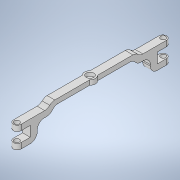
# Autodesk Inventor part: Балка рулевого управления
Saved by Autodesk Inventor 2020 (Build 240168000, 168)
## iProperties
Created: 2021-03-21
Part Number: Балка рулевого управления
Material: Типовые
Document SubType Name: Modeling
Designer: Антон
Density: 1 g/cm^3
Appearance: По умолчанию
Author: Антон
Autodesk Inventor part; units mm, degrees
ref_plane "YZ Plane" through (0, 0, 0) normal (1, 0, 0) x (0, 1, 0)
ref_plane "XZ Plane" through (0, 0, 0) normal (0, 1, 0) x (-1, 0, 0)
ref_plane "XY Plane" through (0, 0, 0) normal (0, 0, 1) x (1, 0, 0)
sketch "Эскиз1" plane through (0, 0, 0) normal (0, 1, 0) x (-1, 0, 0)
  line L0 (0, 0) -> (5.5, 0)
  line L1 (5.5, 0) -> (5.5, -55.05)
  line L2 (5.5, -55.05) -> (0, -55.05)
  line L3 (0, -55.05) -> (0, 0)
  line L4 (2.75, 0) -> (2.75, -2.5)
  circle A0 centre (2.75, -2.5) radius 1.85
  dimension "d0" = 5.5
  dimension "d1" = 55.05
  dimension "d4" = 2.5
  dimension "d5" = 3.7
  constraints: 10 end point, 2 parallel, 1 centre point, 1 coincident, 1 horizontal, 1 midpoint, 1 perpendicular, 1 vertical
  measures "d0" distance of L1.end L2.end
  measures "d1" distance of L0.end L1.end
  measures "d4" distance of L4.start L4.end
  measures "d5" diameter of A0
extrude "Выдавливание1" add sketch "Эскиз1" along normal blind 4
fillet "Сопряжение1" radius 2.75 2 edges at (0, 2, 0) (-5.5, 2, 0)
sketch "Эскиз2" plane through (0, 4, 0) normal (0, 1, 0) x (1, 0, 0)
  line L0 (0, 2.75) -> (0, 55.05) projected
  line L1 (-5.5, 55.05) -> (0, 55.05)
  line L2 (0, 55.05) -> (0, 9.4)
  line L3 (0, 9.4) -> (-5.5, 9.4)
  line L4 (-5.5, 9.4) -> (-5.5, 55.05)
  point P0 (0, 0)
  dimension "d7" = 45.65
  dimension "d45" = 52.3
  constraints: 8 end point, 2 parallel, 1 horizontal, 1 perpendicular, 1 point on line
  measures "d7" distance of L1.end L2.end
  measures "d45" distance of L0.start L0.end
extrude "Выдавливание2" add sketch "Эскиз2" along normal blind 3.7
mirror "Зеркальное отражение3" about plane through (-2.75, 7.7, -32.225) normal (0, 1, 0)
sketch "Эскиз8" plane through (0, 0, -2.75) normal (1, 0, 0) x (0, 0, -1)
  line L0 (0, 0) -> (52.3, 0) projected
  line L1 (52.3, 0) -> (11.65, 0)
  line L2 (11.65, 0) -> (11.65, 15)
  line L3 (11.65, 15) -> (52.3, 15)
  line L4 (52.3, 15) -> (52.3, 0)
  line L5 (6.65, 4) -> (6.65, 11.4) projected
  line L6 (11.65, 15) -> (21.65, 15)
  line L7 (21.65, 15) -> (21.65, 11)
  line L8 (21.65, 11) -> (11.65, 11)
  line L9 (11.65, 11) -> (11.65, 15)
  point P0 (-2.75, 0)
  dimension "d35" = 40.65
  dimension "d36" = 15
  dimension "d52" = 45.65
  dimension "d60" = 10
  dimension "d61" = 4
  constraints: 14 end point, 3 horizontal, 3 parallel, 2 perpendicular, 3 other
  measures "d35" distance of L2.end L4.start
  measures "d36" distance of L1.end L2.end
  measures "d52" distance between parallel lines of L4 L5
  measures "d60" distance of L7.end L8.end
  measures "d61" distance of L6.end L7.end
extrude "Выдавливание6" cut sketch "Эскиз8" against normal through all contours L2 L8 L7 L3 L4 L0
sketch "Эскиз13" plane through (-5.5, 15.4, -55.05) normal (0, 1, 0) x (1, 0, 0)
  line L0 (0, 0) -> (0, -30.65) projected
  line L1 (5.5, 0) -> (0, 0) projected
  line L2 (5.5, -30.65) -> (5.5, 0) projected
  line L3 (5.5, -30.65) -> (0, -30.65) projected
  point P0 (5.5, -55.05)
extrude "Выдавливание11" add sketch "Эскиз13" along normal blind 3
mirror "Зеркальное отражение6" about plane through (0, 0, -55.05) normal (0, 0, -1)
fillet "Сопряжение5" radius 5 12 edges at (-2.75, 0, -14.4) (-2.75, 0, -95.7) (-2.75, 11, -14.4) (-2.75, 11, -24.4) (-2.75, 15, -24.4) (-2.75, 11, -95.7) (-2.75, 11, -85.7) (-2.75, 15, -85.7) (-2.75, 18.4, -24.4) (-2.75, 18.4, -85.7) (-2.75, 15.4, -24.4) (-2.75, 15.4, -85.7)
sketch "Эскиз9" plane through (-2.75, 18.4, -2.75) normal (0, 1, 0) x (1, 0, 0)
  line L0 (2.75, 0) -> (2.75, 21.65) projected
  line L1 (2.75, 52.3) -> (-2.75, 52.3)
  line L2 (-2.75, 21.65) -> (-2.75, 0) projected
  circle A0 centre (0, 52.3) radius 4
  point P0 (2.75, -2.75)
  point P1 (2.75, 104.6)
  point P2 (-2.75, 104.6)
  point P3 (-2.75, 0)
  point P4 (60.3162, 64.5588)
  point P5 (-2.1213, 2.1213)
  point P6 (2.75, 11.65)
  point P7 (-2.75, 11.65)
  point P8 (-2.75, 21.65)
  dimension "d46" = 8
  constraints: 2 end point, 1 centre point, 1 midpoint, 1 point on line, 2 other
  measures "d46" diameter of A0
extrude "Выдавливание7" add sketch "Эскиз9" against normal up to surface (3.4 mm away)
sketch "Эскиз10" plane through (-2.75, 18.4, -2.75) normal (0, 1, 0) x (1, 0, 0)
  arc A0 (-2.75, 55.2047) -> (-2.75, 49.3953) centre (0, 52.3) ccw projected
  arc A1 (-2.75, 55.2047) -> (-2.75, 49.3953) centre (0, 52.3) ccw projected
  circle A2 centre (0, 52.3) radius 2.75
  point P0 (2.75, -2.75)
  point P1 (2.75, 49.3953)
  point P2 (2.75, 55.2047)
  dimension "d49" = 5.5
  constraints: 1 centre point, 1 coincident
  measures "d49" diameter of A2
extrude "Выдавливание8" cut sketch "Эскиз10" against normal blind 2.5
